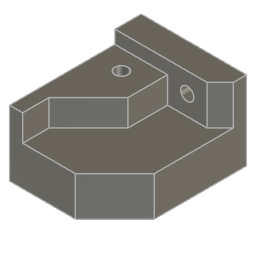
cad1 (Autodesk Fusion 360 design; units mm, degrees)
part number: 2026-02-27-05-04-51-723
Autodesk Fusion 360 part; units mm, degrees
sketch "Sketch1" plane through (0, 0, 0) normal (0, 0, 1) x (1, 0, 0)
  line L0 (0, 0) -> (0, 20)
  line L1 (0, 20) -> (16, 20)
  line L2 (0, 0) -> (6, 0)
  line L3 (0, 0) -> (10, 0)
  line L4 (16, 20) -> (16, 6)
  line L5 (10, 0) -> (16, 6)
  dimension "d1" = 20
  dimension "d2" = 16
  dimension "d3" = 14
  constraint coincident L0.start L2.start
  constraint vertical L0
  constraint perpendicular L0 L1
  constraint perpendicular L0 L2
  constraint perpendicular L0 L3
  constraint perpendicular L1 L4
  measures "d1" distance of L0.start L0.end
  measures "d2" distance of L0.end L1.end
  measures "d3" distance of L1.end L4.end
extrude "Extrude1" add sketch "Sketch1" along normal blind 6
sketch "Sketch2" plane through (0, 0, 6) normal (0, 0, 1) x (-1, 0, 0)
  line L0 (0, 0) -> (-10, 0)
  line L1 (-10, 0) -> (-16, -6)
  line L2 (-16, -6) -> (-16, -20)
  line L3 (-16, -20) -> (0, -20)
  line L4 (0, -20) -> (0, 0)
  line L5 (0, 0) -> (-2, 0)
  line L6 (-2, 0) -> (-2, -4)
  line L7 (0, 0) -> (0, -16)
  line L8 (0, -16) -> (-8, -16)
  line L9 (-8, -16) -> (-8, -10)
  line L10 (-2, -4) -> (-8, -10)
  dimension "d6" = 2
  dimension "d7" = 4
  dimension "d8" = 16
  dimension "d9" = 8
  dimension "d10" = 6
  constraint coincident L0.start L4.end
  constraint perpendicular L4 L5
  constraint perpendicular L5 L6
  constraint perpendicular L3 L7
  constraint perpendicular L7 L8
  constraint perpendicular L8 L9
  measures "d6" distance of L0.start L5.end
  measures "d7" distance of L5.end L6.end
  measures "d8" distance of L0.start L7.end
  measures "d9" distance of L7.end L8.end
  measures "d10" distance of L8.end L9.end
extrude "Extrude2" add sketch "Sketch2" along normal blind 4 contours L0 L4 L5 L6 L7 L8 L9 L10
sketch "Sketch3" plane through (0, 0, 6) normal (0, 0, 1) x (-1, 0, 0)
  line L0 (-2, -4) -> (-2, 0)
  line L1 (-2, 0) -> (-10, 0)
  line L2 (-10, 0) -> (-16, -6)
  line L3 (-16, -6) -> (-16, -20)
  line L4 (-16, -20) -> (0, -20)
  line L5 (0, -20) -> (0, -16)
  line L6 (0, -16) -> (-8, -16)
  line L7 (-8, -16) -> (-8, -10)
  line L8 (-8, -10) -> (-2, -4)
  line L9 (-16, -20) -> (-16, -18)
  line L10 (-8, -16) -> (-14, -16)
  line L11 (-14, -16) -> (-16, -18)
  line L12 (-16, -20) -> (0, -20)
  line L13 (0, -16) -> (0, -20)
  line L14 (0, -16) -> (-8, -16)
  dimension "d13" = 2
  dimension "d14" = 6
  constraint coincident L3.end L4.start
  constraint perpendicular L4 L9
  constraint coincident L6.end L7.start
  constraint perpendicular L3 L10
  constraint coincident L4.end L5.start
  constraint coincident L5.end L6.start
  measures "d13" distance of L3.end L9.end
  measures "d14" distance of L6.end L10.end
extrude "Extrude3" add sketch "Sketch3" along normal blind 6 contours L3 L4 L5 L6 L9 L10 L11 L12 L13 L14
sketch "Sketch4" plane through (0, 0, 10) normal (0, 0, 1) x (-1, 0, 0)
  line L0 (0, 0) -> (-2, 0)
  line L1 (-2, 0) -> (-2, -4)
  line L2 (-2, -4) -> (-8, -10)
  line L3 (-8, -10) -> (-8, -16)
  line L4 (-8, -16) -> (0, -16)
  line L5 (0, -16) -> (0, 0)
  line L6 (-8, -16) -> (-8, -13)
  line L7 (-8, -13) -> (-4, -13)
  dimension "d17" = 4
  constraint coincident L3.end L4.start
  constraint midpoint L3 L6.end
  constraint perpendicular L6 L7
  measures "d17" distance of L6.end L7.end
hole "Hole1" at (4, 13, 10) direction (0, 0, -1) diameter 2 depth 12 tip angle 118
sketch "Sketch5" plane through (0, 16, 0) normal (0, -1, 0) x (1, 0, 0)
  line L0 (0, 10) -> (8, 10)
  line L1 (8, 10) -> (8, 6)
  line L2 (8, 6) -> (14, 6)
  line L3 (14, 6) -> (14, 12)
  line L4 (14, 12) -> (0, 12)
  line L5 (0, 12) -> (0, 10)
  line L6 (14, 12) -> (11, 12)
  line L7 (11, 12) -> (11, 9)
  dimension "d21" = 3
  dimension "d22" = 3
  constraint coincident L3.end L4.start
  constraint perpendicular L3 L6
  constraint perpendicular L6 L7
  measures "d21" distance of L3.end L6.end
  measures "d22" distance of L6.end L7.end
hole "Hole2" at (11, 16, 9) direction (0, 1, 0) diameter 2 depth 12 tip angle 118
